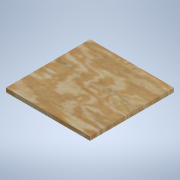
# Autodesk Inventor part: Bottom
Saved by Autodesk Inventor 2021.1 (Build 251245000, 245)
## iProperties
Created: 2020-08-02
Part Number: Bottom
Material: Generic
Document SubType Name: Modeling
Designer: adick
Density: 1 g/cm^3
Appearance: Default
Author: adick
Autodesk Inventor part; units mm, degrees
ref_plane "YZ Plane" through (0, 0, 0) normal (1, 0, 0) x (0, 1, 0)
ref_plane "XZ Plane" through (0, 0, 0) normal (0, 1, 0) x (-1, 0, 0)
ref_plane "XY Plane" through (0, 0, 0) normal (0, 0, 1) x (1, 0, 0)
sketch "Sketch1" plane through (0, 0, 0) normal (0, 0, 1) x (1, 0, 0)
  line L0 (135, 77) -> (135, -77) projected
  line L1 (-135, -77) -> (135, -77)
  line L2 (135, -77) -> (135, -70.65)
  line L3 (-135, -70.65) -> (-135, -77)
  line L4 (-135, -77) -> (135, -77)
  line L5 (135, -77) -> (135, -64.3)
  line L6 (135, -64.3) -> (-135, -64.3)
  line L7 (-135, -64.3) -> (-135, -77)
  point P0 (0, 0)
  point P1 (-135, -7)
  constraints: 14 end point, 3 parallel, 2 horizontal, 2 perpendicular, 3 other
extrude "Extrusion1" add sketch "Sketch1" along normal blind 270
body "Solid1"
